Autodesk Inventor part; units mm, degrees
(part 2 of 4)
  spline S241 degree 2 poles (89.3094, 601.3426) (89.3094, 601.1598) (89.3366, 600.9203) (89.3835, 600.8313) knots 0 0 0 1 2 2 2
  spline S242 degree 2 poles (89.3835, 600.8313) (89.4304, 600.7424) (89.591, 600.6609) (89.7416, 600.6609) knots 0 0 0 1 2 2 2
  spline S243 degree 2 poles (89.7416, 600.6609) (89.8824, 600.6609) (90.2011, 600.8215) (90.3345, 600.9375) knots 0 0 0 1 2 2 2
  line L264 (90.3345, 600.9375) -> (90.3345, 602.6468)
  line L265 (90.3345, 602.6468) -> (90.7198, 602.6468)
  line L266 (90.7198, 602.6468) -> (90.7198, 600.3596)
  spline S244 degree 2 poles (91.8955, 600.3052) (91.6658, 600.3052) (91.2681, 600.4287) (91.1372, 600.4979) knots 0 0 0 1 2 2 2
  line L267 (91.1372, 600.4979) -> (91.1372, 600.9301)
  line L268 (91.1372, 600.9301) -> (91.157, 600.9301)
  spline S245 degree 2 poles (91.157, 600.9301) (91.2064, 600.8906) (91.3397, 600.7968) (91.4509, 600.7449) knots 0 0 0 1 2 2 2
  spline S246 degree 2 poles (91.4509, 600.7449) (91.5472, 600.698) (91.7844, 600.6288) (91.9103, 600.6288) knots 0 0 0 1 2 2 2
  spline S247 degree 2 poles (91.9103, 600.6288) (92.0017, 600.6288) (92.2117, 600.6708) (92.2611, 600.7054) knots 0 0 0 1 2 2 2
  spline S248 degree 2 poles (92.2611, 600.7054) (92.3327, 600.7523) (92.3969, 600.8585) (92.3969, 600.9672) knots 0 0 0 1 2 2 2
  spline S249 degree 2 poles (92.3969, 600.9672) (92.3969, 601.103) (92.2487, 601.2438) (92.0585, 601.2908) knots 0 0 0 1 2 2 2
  spline S250 degree 2 poles (92.0585, 601.2908) (91.9844, 601.3081) (91.7473, 601.3575) (91.646, 601.3846) knots 0 0 0 1 2 2 2
  spline S251 degree 2 poles (91.646, 601.3846) (91.3842, 601.4612) (91.1471, 601.7774) (91.1471, 602.0021) knots 0 0 0 1 2 2 2
  spline S252 degree 2 poles (91.1471, 602.0021) (91.1471, 602.3133) (91.6139, 602.7011) (91.9992, 602.7011) knots 0 0 0 1 2 2 2
  spline S253 degree 2 poles (91.9992, 602.7011) (92.1894, 602.7011) (92.5748, 602.6073) (92.7057, 602.5356) knots 0 0 0 1 2 2 2
  line L269 (92.7057, 602.5356) -> (92.7057, 602.1232)
  line L270 (92.7057, 602.1232) -> (92.6859, 602.1232)
  spline S254 degree 2 poles (92.6859, 602.1232) (92.5377, 602.2417) (92.1771, 602.3776) (91.9918, 602.3776) knots 0 0 0 1 2 2 2
  spline S255 degree 2 poles (91.9918, 602.3776) (91.8016, 602.3776) (91.5398, 602.217) (91.5398, 602.0565) knots 0 0 0 1 2 2 2
  spline S256 degree 2 poles (91.5398, 602.0565) (91.5398, 601.9107) (91.6954, 601.7699) (91.8683, 601.7255) knots 0 0 0 1 2 2 2
  spline S257 degree 2 poles (91.8683, 601.7255) (91.9523, 601.7033) (92.1647, 601.6588) (92.2808, 601.6316) knots 0 0 0 1 2 2 2
  spline S258 degree 2 poles (92.2808, 601.6316) (92.5328, 601.5674) (92.7896, 601.2735) (92.7896, 601.0191) knots 0 0 0 1 2 2 2
  spline S259 degree 2 poles (92.7896, 601.0191) (92.7896, 600.8709) (92.6736, 600.609) (92.5599, 600.5127) knots 0 0 0 1 2 2 2
  spline S260 degree 2 poles (92.5599, 600.5127) (92.4389, 600.4114) (92.1302, 600.3052) (91.8955, 600.3052) knots 0 0 0 1 2 2 2
  spline S261 degree 2 poles (93.7653, 600.3052) (93.5356, 600.3052) (93.1379, 600.4287) (93.007, 600.4979) knots 0 0 0 1 2 2 2
  line L271 (93.007, 600.4979) -> (93.007, 600.9301)
  line L272 (93.007, 600.9301) -> (93.0268, 600.9301)
  spline S262 degree 2 poles (93.0268, 600.9301) (93.0762, 600.8906) (93.2095, 600.7968) (93.3207, 600.7449) knots 0 0 0 1 2 2 2
  spline S263 degree 2 poles (93.3207, 600.7449) (93.417, 600.698) (93.6542, 600.6288) (93.7801, 600.6288) knots 0 0 0 1 2 2 2
  spline S264 degree 2 poles (93.7801, 600.6288) (93.8715, 600.6288) (94.0815, 600.6708) (94.1309, 600.7054) knots 0 0 0 1 2 2 2
  spline S265 degree 2 poles (94.1309, 600.7054) (94.2025, 600.7523) (94.2667, 600.8585) (94.2667, 600.9672) knots 0 0 0 1 2 2 2
  spline S266 degree 2 poles (94.2667, 600.9672) (94.2667, 601.103) (94.1185, 601.2438) (93.9283, 601.2908) knots 0 0 0 1 2 2 2
  spline S267 degree 2 poles (93.9283, 601.2908) (93.8542, 601.3081) (93.6171, 601.3575) (93.5158, 601.3846) knots 0 0 0 1 2 2 2
  spline S268 degree 2 poles (93.5158, 601.3846) (93.254, 601.4612) (93.0169, 601.7774) (93.0169, 602.0021) knots 0 0 0 1 2 2 2
  spline S269 degree 2 poles (93.0169, 602.0021) (93.0169, 602.3133) (93.4837, 602.7011) (93.869, 602.7011) knots 0 0 0 1 2 2 2
  spline S270 degree 2 poles (93.869, 602.7011) (94.0592, 602.7011) (94.4446, 602.6073) (94.5755, 602.5356) knots 0 0 0 1 2 2 2
  line L273 (94.5755, 602.5356) -> (94.5755, 602.1232)
  line L274 (94.5755, 602.1232) -> (94.5557, 602.1232)
  spline S271 degree 2 poles (94.5557, 602.1232) (94.4075, 602.2417) (94.0469, 602.3776) (93.8616, 602.3776) knots 0 0 0 1 2 2 2
  spline S272 degree 2 poles (93.8616, 602.3776) (93.6714, 602.3776) (93.4096, 602.217) (93.4096, 602.0565) knots 0 0 0 1 2 2 2
  spline S273 degree 2 poles (93.4096, 602.0565) (93.4096, 601.9107) (93.5652, 601.7699) (93.7381, 601.7255) knots 0 0 0 1 2 2 2
  spline S274 degree 2 poles (93.7381, 601.7255) (93.8221, 601.7033) (94.0345, 601.6588) (94.1506, 601.6316) knots 0 0 0 1 2 2 2
  spline S275 degree 2 poles (94.1506, 601.6316) (94.4026, 601.5674) (94.6594, 601.2735) (94.6594, 601.0191) knots 0 0 0 1 2 2 2
  spline S276 degree 2 poles (94.6594, 601.0191) (94.6594, 600.8709) (94.5434, 600.609) (94.4297, 600.5127) knots 0 0 0 1 2 2 2
  spline S277 degree 2 poles (94.4297, 600.5127) (94.3087, 600.4114) (94, 600.3052) (93.7653, 600.3052) knots 0 0 0 1 2 2 2
  line L275 (95.4103, 600.3596) -> (95.025, 600.3596)
  line L276 (95.025, 600.3596) -> (95.025, 602.6468)
  line L277 (95.025, 602.6468) -> (95.4103, 602.6468)
  line L278 (95.4103, 602.6468) -> (95.4103, 600.3596)
  line L279 (95.4375, 603.0272) -> (95.0003, 603.0272)
  line L280 (95.0003, 603.0272) -> (95.0003, 603.4273)
  line L281 (95.0003, 603.4273) -> (95.4375, 603.4273)
  line L282 (95.4375, 603.4273) -> (95.4375, 603.0272)
  spline S278 degree 2 poles (97.8557, 601.5032) (97.8557, 600.9252) (97.2999, 600.2953) (96.8355, 600.2953) knots 0 0 0 1 2 2 2
  spline S279 degree 2 poles (96.8355, 600.2953) (96.3588, 600.2953) (95.8129, 600.945) (95.8129, 601.5032) knots 0 0 0 1 2 2 2
  spline S280 degree 2 poles (95.8129, 601.5032) (95.8129, 602.0762) (96.3761, 602.711) (96.8355, 602.711) knots 0 0 0 1 2 2 2
  spline S281 degree 2 poles (96.8355, 602.711) (97.2999, 602.711) (97.8557, 602.0787) (97.8557, 601.5032) knots 0 0 0 1 2 2 2
  spline S282 degree 2 poles (97.458, 601.5032) (97.458, 601.9478) (97.1344, 602.38) (96.8355, 602.38) knots 0 0 0 1 2 2 2
  spline S283 degree 2 poles (96.8355, 602.38) (96.5367, 602.38) (96.2106, 601.9478) (96.2106, 601.5032) knots 0 0 0 1 2 2 2
  spline S284 degree 2 poles (96.2106, 601.5032) (96.2106, 601.0709) (96.5367, 600.6263) (96.8355, 600.6263) knots 0 0 0 1 2 2 2
  spline S285 degree 2 poles (96.8355, 600.6263) (97.1319, 600.6263) (97.458, 601.0635) (97.458, 601.5032) knots 0 0 0 1 2 2 2
  line L283 (100.0466, 600.3596) -> (99.6612, 600.3596)
  line L284 (99.6612, 600.3596) -> (99.6612, 601.6637)
  spline S286 degree 2 poles (99.6612, 601.6637) (99.6612, 601.8218) (99.6316, 602.0935) (99.5871, 602.175) knots 0 0 0 1 2 2 2
  spline S287 degree 2 poles (99.5871, 602.175) (99.5402, 602.2615) (99.3722, 602.3455) (99.229, 602.3455) knots 0 0 0 1 2 2 2
  spline S288 degree 2 poles (99.229, 602.3455) (99.0857, 602.3455) (98.7819, 602.1923) (98.6362, 602.0688) knots 0 0 0 1 2 2 2
  line L285 (98.6362, 602.0688) -> (98.6362, 600.3596)
  line L286 (98.6362, 600.3596) -> (98.2509, 600.3596)
  line L287 (98.2509, 600.3596) -> (98.2509, 602.6468)
  line L288 (98.2509, 602.6468) -> (98.6362, 602.6468)
  line L289 (98.6362, 602.6468) -> (98.6362, 602.3924)
  spline S289 degree 2 poles (98.6362, 602.3924) (98.8091, 602.548) (99.1425, 602.711) (99.3302, 602.711) knots 0 0 0 1 2 2 2
  spline S290 degree 2 poles (99.3302, 602.711) (99.6662, 602.711) (100.0466, 602.2664) (100.0466, 601.844) knots 0 0 0 1 2 2 2
  line L290 (100.0466, 601.844) -> (100.0466, 600.3596)
  line L291 (101.6471, 601.5081) -> (100.4936, 601.5081)
  line L292 (100.4936, 601.5081) -> (100.4936, 601.8786)
  line L293 (100.4936, 601.8786) -> (101.6471, 601.8786)
  line L294 (101.6471, 601.8786) -> (101.6471, 601.5081)
  line L295 (104.7519, 600.3596) -> (104.3469, 600.3596)
  line L296 (104.3469, 600.3596) -> (104.3469, 602.9852)
  line L297 (104.3469, 602.9852) -> (103.5515, 601.1994)
  line L298 (103.5515, 601.1994) -> (103.3045, 601.1994)
  line L299 (103.3045, 601.1994) -> (102.5166, 602.9852)
  line L300 (102.5166, 602.9852) -> (102.5166, 600.3596)
  line L301 (102.5166, 600.3596) -> (102.1387, 600.3596)
  line L302 (102.1387, 600.3596) -> (102.1387, 603.4076)
  line L303 (102.1387, 603.4076) -> (102.6919, 603.4076)
  line L304 (102.6919, 603.4076) -> (103.4527, 601.7107)
  line L305 (103.4527, 601.7107) -> (104.1888, 603.4076)
  line L306 (104.1888, 603.4076) -> (104.7519, 603.4076)
  line L307 (104.7519, 603.4076) -> (104.7519, 600.3596)
  spline S291 degree 2 poles (106.6143, 600.6016) (106.5674, 600.567) (106.4093, 600.4435) (106.3352, 600.4065) knots 0 0 0 1 2 2 2
  spline S292 degree 2 poles (106.3352, 600.4065) (106.2339, 600.3522) (106.0438, 600.2953) (105.8709, 600.2953) knots 0 0 0 1 2 2 2
  spline S293 degree 2 poles (105.8709, 600.2953) (105.7301, 600.2953) (105.4757, 600.4016) (105.3793, 600.4979) knots 0 0 0 1 2 2 2
  spline S294 degree 2 poles (105.3793, 600.4979) (105.2879, 600.5917) (105.1768, 600.8684) (105.1768, 601.0215) knots 0 0 0 1 2 2 2
  spline S295 degree 2 poles (105.1768, 601.0215) (105.1768, 601.2587) (105.3768, 601.5946) (105.5942, 601.6909) knots 0 0 0 1 2 2 2
  spline S296 degree 2 poles (105.5942, 601.6909) (105.7869, 601.7798) (106.3105, 601.8465) (106.6143, 601.8638) knots 0 0 0 1 2 2 2
  line L308 (106.6143, 601.8638) -> (106.6143, 601.9379)
  spline S297 degree 2 poles (106.6143, 601.9379) (106.6143, 602.0713) (106.5328, 602.2368) (106.4587, 602.2837) knots 0 0 0 1 2 2 2
  spline S298 degree 2 poles (106.4587, 602.2837) (106.3846, 602.3306) (106.1722, 602.3603) (106.0586, 602.3603) knots 0 0 0 1 2 2 2
  spline S299 degree 2 poles (106.0586, 602.3603) (105.9252, 602.3603) (105.5646, 602.2812) (105.3843, 602.2047) knots 0 0 0 1 2 2 2
  line L309 (105.3843, 602.2047) -> (105.362, 602.2047)
  line L310 (105.362, 602.2047) -> (105.362, 602.5974)
  spline S300 degree 2 poles (105.362, 602.5974) (105.4682, 602.627) (105.8659, 602.7011) (106.061, 602.7011) knots 0 0 0 1 2 2 2
  spline S301 degree 2 poles (106.061, 602.7011) (106.2982, 602.7011) (106.6217, 602.627) (106.7502, 602.5307) knots 0 0 0 1 2 2 2
  spline S302 degree 2 poles (106.7502, 602.5307) (106.8761, 602.4368) (106.9997, 602.138) (106.9997, 601.9231) knots 0 0 0 1 2 2 2
  line L311 (106.9997, 601.9231) -> (106.9997, 600.3596)
  line L312 (106.9997, 600.3596) -> (106.6143, 600.3596)
  line L313 (106.6143, 600.3596) -> (106.6143, 600.6016)
  line L314 (106.6143, 600.9227) -> (106.6143, 601.5575)
  spline S303 degree 2 poles (106.6143, 601.5575) (106.476, 601.5452) (106.0586, 601.5032) (105.9277, 601.4637) knots 0 0 0 1 2 2 2
  spline S304 degree 2 poles (105.9277, 601.4637) (105.7745, 601.4167) (105.5745, 601.2216) (105.5745, 601.0487) knots 0 0 0 1 2 2 2
  spline S305 degree 2 poles (105.5745, 601.0487) (105.5745, 600.8511) (105.7968, 600.651) (106.0092, 600.651) knots 0 0 0 1 2 2 2
  spline S306 degree 2 poles (106.0092, 600.651) (106.1895, 600.651) (106.4859, 600.8066) (106.6143, 600.9227) knots 0 0 0 1 2 2 2
  line L315 (108.7534, 602.2343) -> (108.7336, 602.2343)
  spline S307 degree 2 poles (108.7336, 602.2343) (108.6891, 602.2467) (108.5928, 602.2516) (108.5261, 602.2516) knots 0 0 0 1 2 2 2
  spline S308 degree 2 poles (108.5261, 602.2516) (108.3705, 602.2516) (108.0642, 602.1157) (107.9259, 601.9824) knots 0 0 0 1 2 2 2
  line L316 (107.9259, 601.9824) -> (107.9259, 600.3596)
  line L317 (107.9259, 600.3596) -> (107.5406, 600.3596)
  line L318 (107.5406, 600.3596) -> (107.5406, 602.6468)
  line L319 (107.5406, 602.6468) -> (107.9259, 602.6468)
  line L320 (107.9259, 602.6468) -> (107.9259, 602.3059)
  spline S309 degree 2 poles (107.9259, 602.3059) (108.1359, 602.4937) (108.4495, 602.6468) (108.5978, 602.6468) knots 0 0 0 1 2 2 2
  spline S310 degree 2 poles (108.5978, 602.6468) (108.657, 602.6468) (108.7163, 602.6419) (108.7534, 602.6344) knots 0 0 0 1 2 2 2
  line L321 (108.7534, 602.6344) -> (108.7534, 602.2343)
  spline S311 degree 2 poles (109.9612, 600.3077) (109.7241, 600.3077) (109.3313, 600.4534) (109.1906, 600.6016) knots 0 0 0 1 2 2 2
  spline S312 degree 2 poles (109.1906, 600.6016) (109.0498, 600.7474) (108.8942, 601.1969) (108.8942, 601.4982) knots 0 0 0 1 2 2 2
  spline S313 degree 2 poles (108.8942, 601.4982) (108.8942, 601.7996) (109.0547, 602.2392) (109.1906, 602.3874) knots 0 0 0 1 2 2 2
  spline S314 degree 2 poles (109.1906, 602.3874) (109.3264, 602.5381) (109.729, 602.6987) (109.9612, 602.6987) knots 0 0 0 1 2 2 2
  spline S315 degree 2 poles (109.9612, 602.6987) (110.1489, 602.6987) (110.4997, 602.5925) (110.6355, 602.5233) knots 0 0 0 1 2 2 2
  line L322 (110.6355, 602.5233) -> (110.6355, 602.091)
  line L323 (110.6355, 602.091) -> (110.6133, 602.091)
  spline S316 degree 2 poles (110.6133, 602.091) (110.5713, 602.1256) (110.4429, 602.2145) (110.3515, 602.2615) knots 0 0 0 1 2 2 2
  spline S317 degree 2 poles (110.3515, 602.2615) (110.27, 602.301) (110.0526, 602.3627) (109.9538, 602.3627) knots 0 0 0 1 2 2 2
  spline S318 degree 2 poles (109.9538, 602.3627) (109.6549, 602.3627) (109.2918, 601.9107) (109.2918, 601.4982) knots 0 0 0 1 2 2 2
  spline S319 degree 2 poles (109.2918, 601.4982) (109.2918, 601.0956) (109.6426, 600.6436) (109.9538, 600.6436) knots 0 0 0 1 2 2 2
  spline S320 degree 2 poles (109.9538, 600.6436) (110.1415, 600.6436) (110.4824, 600.7992) (110.6133, 600.9203) knots 0 0 0 1 2 2 2
  line L324 (110.6133, 600.9203) -> (110.6355, 600.9203)
  line L325 (110.6355, 600.9203) -> (110.6355, 600.488)
  spline S321 degree 2 poles (110.6355, 600.488) (110.5787, 600.4608) (110.4058, 600.3843) (110.3366, 600.367) knots 0 0 0 1 2 2 2
  spline S322 degree 2 poles (110.3366, 600.367) (110.2378, 600.3373) (110.0822, 600.3077) (109.9612, 600.3077) knots 0 0 0 1 2 2 2
  line L326 (112.782, 600.3596) -> (112.3966, 600.3596)
  line L327 (112.3966, 600.3596) -> (112.3966, 601.6637)
  spline S323 degree 2 poles (112.3966, 601.6637) (112.3966, 601.8218) (112.367, 602.0935) (112.3225, 602.175) knots 0 0 0 1 2 2 2
  spline S324 degree 2 poles (112.3225, 602.175) (112.2756, 602.2615) (112.1076, 602.3455) (111.9644, 602.3455) knots 0 0 0 1 2 2 2
  spline S325 degree 2 poles (111.9644, 602.3455) (111.8211, 602.3455) (111.5173, 602.1923) (111.3716, 602.0688) knots 0 0 0 1 2 2 2
  line L328 (111.3716, 602.0688) -> (111.3716, 600.3596)
  line L329 (111.3716, 600.3596) -> (110.9863, 600.3596)
  line L330 (110.9863, 600.3596) -> (110.9863, 603.5434)
  line L331 (110.9863, 603.5434) -> (111.3716, 603.5434)
  line L332 (111.3716, 603.5434) -> (111.3716, 602.3924)
  spline S326 degree 2 poles (111.3716, 602.3924) (111.5445, 602.548) (111.8779, 602.711) (112.0657, 602.711) knots 0 0 0 1 2 2 2
  spline S327 degree 2 poles (112.0657, 602.711) (112.4016, 602.711) (112.782, 602.2664) (112.782, 601.844) knots 0 0 0 1 2 2 2
  line L333 (112.782, 601.844) -> (112.782, 600.3596)
  line L334 (113.7156, 600.3596) -> (113.3303, 600.3596)
  line L335 (113.3303, 600.3596) -> (113.3303, 602.6468)
  line L336 (113.3303, 602.6468) -> (113.7156, 602.6468)
  line L337 (113.7156, 602.6468) -> (113.7156, 600.3596)
  line L338 (113.7428, 603.0272) -> (113.3056, 603.0272)
  line L339 (113.3056, 603.0272) -> (113.3056, 603.4273)
  line L340 (113.3056, 603.4273) -> (113.7428, 603.4273)
  line L341 (113.7428, 603.4273) -> (113.7428, 603.0272)
  line L342 (116.077, 600.3596) -> (115.6916, 600.3596)
  line L343 (115.6916, 600.3596) -> (115.6916, 601.6637)
  spline S328 degree 2 poles (115.6916, 601.6637) (115.6916, 601.8218) (115.662, 602.0935) (115.6175, 602.175) knots 0 0 0 1 2 2 2
  spline S329 degree 2 poles (115.6175, 602.175) (115.5706, 602.2615) (115.4026, 602.3455) (115.2594, 602.3455) knots 0 0 0 1 2 2 2
  spline S330 degree 2 poles (115.2594, 602.3455) (115.1161, 602.3455) (114.8123, 602.1923) (114.6666, 602.0688) knots 0 0 0 1 2 2 2
  line L344 (114.6666, 602.0688) -> (114.6666, 600.3596)
  line L345 (114.6666, 600.3596) -> (114.2813, 600.3596)
  line L346 (114.2813, 600.3596) -> (114.2813, 602.6468)
  line L347 (114.2813, 602.6468) -> (114.6666, 602.6468)
  line L348 (114.6666, 602.6468) -> (114.6666, 602.3924)
  spline S331 degree 2 poles (114.6666, 602.3924) (114.8395, 602.548) (115.1729, 602.711) (115.3607, 602.711) knots 0 0 0 1 2 2 2
  spline S332 degree 2 poles (115.3607, 602.711) (115.6966, 602.711) (116.077, 602.2664) (116.077, 601.844) knots 0 0 0 1 2 2 2
  line L349 (116.077, 601.844) -> (116.077, 600.3596)
  spline S333 degree 2 poles (116.6994, 599.994) (116.7389, 599.9767) (116.8896, 599.9224) (116.9859, 599.9001) knots 0 0 0 1 2 2 2
  spline S334 degree 2 poles (116.9859, 599.9001) (117.0921, 599.873) (117.2724, 599.8409) (117.3787, 599.8409) knots 0 0 0 1 2 2 2
  spline S335 degree 2 poles (117.3787, 599.8409) (117.5565, 599.8409) (117.8035, 599.9347) (117.8727, 600.0187) knots 0 0 0 1 2 2 2
  spline S336 degree 2 poles (117.8727, 600.0187) (117.9394, 600.1027) (117.9912, 600.3225) (117.9912, 600.4633) knots 0 0 0 1 2 2 2
  line L350 (117.9912, 600.4633) -> (117.9912, 600.6634)
  spline S337 degree 2 poles (117.9912, 600.6634) (117.8356, 600.5275) (117.5367, 600.3991) (117.312, 600.3991) knots 0 0 0 1 2 2 2
  spline S338 degree 2 poles (117.312, 600.3991) (116.9217, 600.3991) (116.4598, 600.9795) (116.4598, 601.5254) knots 0 0 0 1 2 2 2
  spline S339 degree 2 poles (116.4598, 601.5254) (116.4598, 601.8095) (116.6204, 602.2491) (116.7537, 602.4047) knots 0 0 0 1 2 2 2
  spline S340 degree 2 poles (116.7537, 602.4047) (116.8822, 602.5505) (117.2354, 602.711) (117.4231, 602.711) knots 0 0 0 1 2 2 2
  spline S341 degree 2 poles (117.4231, 602.711) (117.601, 602.711) (117.8603, 602.627) (117.9912, 602.5505) knots 0 0 0 1 2 2 2
  line L351 (117.9912, 602.5505) -> (118.0135, 602.6468)
  line L352 (118.0135, 602.6468) -> (118.3765, 602.6468)
  line L353 (118.3765, 602.6468) -> (118.3765, 600.6214)
  spline S342 degree 2 poles (118.3765, 600.6214) (118.3765, 600.0385) (117.8702, 599.4951) (117.349, 599.4951) knots 0 0 0 1 2 2 2
  spline S343 degree 2 poles (117.349, 599.4951) (117.1811, 599.4951) (116.8303, 599.5494) (116.6796, 599.5939) knots 0 0 0 1 2 2 2
  line L354 (116.6796, 599.5939) -> (116.6796, 599.994)
  line L355 (116.6796, 599.994) -> (116.6994, 599.994)
  line L356 (117.9912, 600.9795) -> (117.9912, 602.2368)
  spline S344 degree 2 poles (117.9912, 602.2368) (117.848, 602.3059) (117.6059, 602.3652) (117.4849, 602.3652) knots 0 0 0 1 2 2 2
  spline S345 degree 2 poles (117.4849, 602.3652) (117.1934, 602.3652) (116.8575, 601.9354) (116.8575, 601.5328) knots 0 0 0 1 2 2 2
  spline S346 degree 2 poles (116.8575, 601.5328) (116.8575, 601.1524) (117.1119, 600.7548) (117.3984, 600.7548) knots 0 0 0 1 2 2 2
  spline S347 degree 2 poles (117.3984, 600.7548) (117.5491, 600.7548) (117.8653, 600.8733) (117.9912, 600.9795) knots 0 0 0 1 2 2 2
  line L357 (119.9944, 601.5081) -> (118.8409, 601.5081)
  line L358 (118.8409, 601.5081) -> (118.8409, 601.8786)
  line L359 (118.8409, 601.8786) -> (119.9944, 601.8786)
  line L360 (119.9944, 601.8786) -> (119.9944, 601.5081)
  spline S348 degree 2 poles (121.6765, 600.3052) (121.3801, 600.3052) (120.8787, 600.5053) (120.6959, 600.7054) knots 0 0 0 1 2 2 2
  spline S349 degree 2 poles (120.6959, 600.7054) (120.5131, 600.903) (120.313, 601.4958) (120.313, 601.8811) knots 0 0 0 1 2 2 2
  spline S350 degree 2 poles (120.313, 601.8811) (120.313, 602.2639) (120.5082, 602.8321) (120.6934, 603.042) knots 0 0 0 1 2 2 2
  spline S351 degree 2 poles (120.6934, 603.042) (120.8762, 603.247) (121.3751, 603.4619) (121.6839, 603.4619) knots 0 0 0 1 2 2 2
  spline S352 degree 2 poles (121.6839, 603.4619) (121.837, 603.4619) (122.1063, 603.4174) (122.2199, 603.3829) knots 0 0 0 1 2 2 2
  spline S353 degree 2 poles (122.2199, 603.3829) (122.3187, 603.3508) (122.5237, 603.2594) (122.625, 603.205) knots 0 0 0 1 2 2 2
  line L361 (122.625, 603.205) -> (122.625, 602.716)
  line L362 (122.625, 602.716) -> (122.5929, 602.716)
  spline S354 degree 2 poles (122.5929, 602.716) (122.5385, 602.7654) (122.3706, 602.9037) (122.2495, 602.9704) knots 0 0 0 1 2 2 2
  spline S355 degree 2 poles (122.2495, 602.9704) (122.1334, 603.0346) (121.8593, 603.1161) (121.6814, 603.1161) knots 0 0 0 1 2 2 2
  spline S356 degree 2 poles (121.6814, 603.1161) (121.4863, 603.1161) (121.138, 602.9556) (121.0071, 602.8024) knots 0 0 0 1 2 2 2
  spline S357 degree 2 poles (121.0071, 602.8024) (120.8787, 602.6468) (120.7354, 602.175) (120.7354, 601.8811) knots 0 0 0 1 2 2 2
  spline S358 degree 2 poles (120.7354, 601.8811) (120.7354, 601.5674) (120.8861, 601.1154) (121.017, 600.9598) knots 0 0 0 1 2 2 2
  spline S359 degree 2 poles (121.017, 600.9598) (121.1454, 600.8091) (121.4888, 600.656) (121.6814, 600.656) knots 0 0 0 1 2 2 2
  spline S360 degree 2 poles (121.6814, 600.656) (121.8568, 600.656) (122.1557, 600.7424) (122.2718, 600.8066) knots 0 0 0 1 2 2 2
  spline S361 degree 2 poles (122.2718, 600.8066) (122.3829, 600.8709) (122.5484, 601.0042) (122.5953, 601.0512) knots 0 0 0 1 2 2 2
  line L363 (122.5953, 601.0512) -> (122.625, 601.0512)
  line L364 (122.625, 601.0512) -> (122.625, 600.567)
  spline S362 degree 2 poles (122.625, 600.567) (122.5237, 600.5201) (122.3459, 600.4337) (122.2199, 600.3941) knots 0 0 0 1 2 2 2
  spline S363 degree 2 poles (122.2199, 600.3941) (122.0865, 600.3497) (121.8593, 600.3052) (121.6765, 600.3052) knots 0 0 0 1 2 2 2
  spline S364 degree 2 poles (124.2478, 600.6016) (124.2008, 600.567) (124.0428, 600.4435) (123.9687, 600.4065) knots 0 0 0 1 2 2 2
  spline S365 degree 2 poles (123.9687, 600.4065) (123.8674, 600.3522) (123.6772, 600.2953) (123.5043, 600.2953) knots 0 0 0 1 2 2 2
  spline S366 degree 2 poles (123.5043, 600.2953) (123.3635, 600.2953) (123.1091, 600.4016) (123.0128, 600.4979) knots 0 0 0 1 2 2 2
  spline S367 degree 2 poles (123.0128, 600.4979) (122.9214, 600.5917) (122.8102, 600.8684) (122.8102, 601.0215) knots 0 0 0 1 2 2 2
  spline S368 degree 2 poles (122.8102, 601.0215) (122.8102, 601.2587) (123.0103, 601.5946) (123.2277, 601.6909) knots 0 0 0 1 2 2 2
  spline S369 degree 2 poles (123.2277, 601.6909) (123.4203, 601.7798) (123.944, 601.8465) (124.2478, 601.8638) knots 0 0 0 1 2 2 2
  line L365 (124.2478, 601.8638) -> (124.2478, 601.9379)
  spline S370 degree 2 poles (124.2478, 601.9379) (124.2478, 602.0713) (124.1663, 602.2368) (124.0922, 602.2837) knots 0 0 0 1 2 2 2
  spline S371 degree 2 poles (124.0922, 602.2837) (124.0181, 602.3306) (123.8056, 602.3603) (123.692, 602.3603) knots 0 0 0 1 2 2 2
  spline S372 degree 2 poles (123.692, 602.3603) (123.5586, 602.3603) (123.198, 602.2812) (123.0177, 602.2047) knots 0 0 0 1 2 2 2
  line L366 (123.0177, 602.2047) -> (122.9955, 602.2047)
  line L367 (122.9955, 602.2047) -> (122.9955, 602.5974)
  spline S373 degree 2 poles (122.9955, 602.5974) (123.1017, 602.627) (123.4994, 602.7011) (123.6945, 602.7011) knots 0 0 0 1 2 2 2
  spline S374 degree 2 poles (123.6945, 602.7011) (123.9316, 602.7011) (124.2552, 602.627) (124.3836, 602.5307) knots 0 0 0 1 2 2 2
  spline S375 degree 2 poles (124.3836, 602.5307) (124.5096, 602.4368) (124.6331, 602.138) (124.6331, 601.9231) knots 0 0 0 1 2 2 2
  line L368 (124.6331, 601.9231) -> (124.6331, 600.3596)
  line L369 (124.6331, 600.3596) -> (124.2478, 600.3596)
  line L370 (124.2478, 600.3596) -> (124.2478, 600.6016)
  line L371 (124.2478, 600.9227) -> (124.2478, 601.5575)
  spline S376 degree 2 poles (124.2478, 601.5575) (124.1095, 601.5452) (123.692, 601.5032) (123.5611, 601.4637) knots 0 0 0 1 2 2 2
  spline S377 degree 2 poles (123.5611, 601.4637) (123.408, 601.4167) (123.2079, 601.2216) (123.2079, 601.0487) knots 0 0 0 1 2 2 2
  spline S378 degree 2 poles (123.2079, 601.0487) (123.2079, 600.8511) (123.4302, 600.651) (123.6426, 600.651) knots 0 0 0 1 2 2 2
  spline S379 degree 2 poles (123.6426, 600.651) (123.8229, 600.651) (124.1193, 600.8066) (124.2478, 600.9227) knots 0 0 0 1 2 2 2
  line L372 (126.3868, 602.2343) -> (126.367, 602.2343)
  spline S380 degree 2 poles (126.367, 602.2343) (126.3226, 602.2467) (126.2263, 602.2516) (126.1596, 602.2516) knots 0 0 0 1 2 2 2
  spline S381 degree 2 poles (126.1596, 602.2516) (126.004, 602.2516) (125.6977, 602.1157) (125.5594, 601.9824) knots 0 0 0 1 2 2 2
  line L373 (125.5594, 601.9824) -> (125.5594, 600.3596)
  line L374 (125.5594, 600.3596) -> (125.174, 600.3596)
  line L375 (125.174, 600.3596) -> (125.174, 602.6468)
  line L376 (125.174, 602.6468) -> (125.5594, 602.6468)
  line L377 (125.5594, 602.6468) -> (125.5594, 602.3059)
  spline S382 degree 2 poles (125.5594, 602.3059) (125.7693, 602.4937) (126.083, 602.6468) (126.2312, 602.6468) knots 0 0 0 1 2 2 2
  spline S383 degree 2 poles (126.2312, 602.6468) (126.2905, 602.6468) (126.3498, 602.6419) (126.3868, 602.6344) knots 0 0 0 1 2 2 2
  line L378 (126.3868, 602.6344) -> (126.3868, 602.2343)
  line L379 (127.8985, 602.2343) -> (127.8787, 602.2343)
  spline S384 degree 2 poles (127.8787, 602.2343) (127.8342, 602.2467) (127.7379, 602.2516) (127.6712, 602.2516) knots 0 0 0 1 2 2 2
  spline S385 degree 2 poles (127.6712, 602.2516) (127.5156, 602.2516) (127.2093, 602.1157) (127.071, 601.9824) knots 0 0 0 1 2 2 2
  line L380 (127.071, 601.9824) -> (127.071, 600.3596)
  line L381 (127.071, 600.3596) -> (126.6857, 600.3596)
  line L382 (126.6857, 600.3596) -> (126.6857, 602.6468)
  line L383 (126.6857, 602.6468) -> (127.071, 602.6468)
  line L384 (127.071, 602.6468) -> (127.071, 602.3059)
  spline S386 degree 2 poles (127.071, 602.3059) (127.281, 602.4937) (127.5946, 602.6468) (127.7428, 602.6468) knots 0 0 0 1 2 2 2
  spline S387 degree 2 poles (127.7428, 602.6468) (127.8021, 602.6468) (127.8614, 602.6419) (127.8985, 602.6344) knots 0 0 0 1 2 2 2
  line L385 (127.8985, 602.6344) -> (127.8985, 602.2343)
  line L386 (128.5901, 600.3596) -> (128.2047, 600.3596)
  line L387 (128.2047, 600.3596) -> (128.2047, 602.6468)
  line L388 (128.2047, 602.6468) -> (128.5901, 602.6468)
  line L389 (128.5901, 602.6468) -> (128.5901, 600.3596)
  line L390 (128.6172, 603.0272) -> (128.18, 603.0272)
  line L391 (128.18, 603.0272) -> (128.18, 603.4273)
  line L392 (128.18, 603.4273) -> (128.6172, 603.4273)
  line L393 (128.6172, 603.4273) -> (128.6172, 603.0272)
  spline S388 degree 2 poles (130.1486, 600.3077) (129.6003, 600.3077) (128.9976, 600.9227) (128.9976, 601.4908) knots 0 0 0 1 2 2 2
  spline S389 degree 2 poles (128.9976, 601.4908) (128.9976, 602.0491) (129.583, 602.711) (130.0548, 602.711) knots 0 0 0 1 2 2 2
  spline S390 degree 2 poles (130.0548, 602.711) (130.2672, 602.711) (130.5957, 602.5875) (130.7167, 602.4566) knots 0 0 0 1 2 2 2
  spline S391 degree 2 poles (130.7167, 602.4566) (130.8402, 602.3257) (130.9712, 601.9478) (130.9712, 601.6736) knots 0 0 0 1 2 2 2
  line L394 (130.9712, 601.6736) -> (130.9712, 601.4637)
  line L395 (130.9712, 601.4637) -> (129.3879, 601.4637)
  spline S392 degree 2 poles (129.3879, 601.4637) (129.3879, 601.066) (129.788, 600.6436) (130.1437, 600.6436) knots 0 0 0 1 2 2 2
  spline S393 degree 2 poles (130.1437, 600.6436) (130.2697, 600.6436) (130.5142, 600.7004) (130.613, 600.7449) knots 0 0 0 1 2 2 2
  spline S394 degree 2 poles (130.613, 600.7449) (130.7167, 600.7943) (130.86, 600.8807) (130.9069, 600.9203) knots 0 0 0 1 2 2 2
  line L396 (130.9069, 600.9203) -> (130.9292, 600.9203)
  line L397 (130.9292, 600.9203) -> (130.9292, 600.5004)
  spline S395 degree 2 poles (130.9292, 600.5004) (130.8625, 600.4732) (130.6599, 600.3941) (130.5809, 600.3719) knots 0 0 0 1 2 2 2
  spline S396 degree 2 poles (130.5809, 600.3719) (130.4697, 600.3398) (130.287, 600.3077) (130.1486, 600.3077) knots 0 0 0 1 2 2 2
  spline S397 degree 2 poles (130.5957, 601.7576) (130.5908, 601.9132) (130.5266, 602.1404) (130.4648, 602.217) knots 0 0 0 1 2 2 2
  spline S398 degree 2 poles (130.4648, 602.217) (130.3981, 602.3035) (130.1882, 602.3949) (130.0326, 602.3949) knots 0 0 0 1 2 2 2
  spline S399 degree 2 poles (130.0326, 602.3949) (129.8794, 602.3949) (129.6645, 602.3035) (129.5756, 602.2145) knots 0 0 0 1 2 2 2
  spline S400 degree 2 poles (129.5756, 602.2145) (129.4891, 602.1232) (129.4002, 601.9033) (129.3879, 601.7576) knots 0 0 0 1 2 2 2
  line L398 (129.3879, 601.7576) -> (130.5957, 601.7576)
  line L399 (132.5742, 602.2343) -> (132.5544, 602.2343)
  spline S401 degree 2 poles (132.5544, 602.2343) (132.51, 602.2467) (132.4136, 602.2516) (132.347, 602.2516) knots 0 0 0 1 2 2 2
  spline S402 degree 2 poles (132.347, 602.2516) (132.1913, 602.2516) (131.8851, 602.1157) (131.7467, 601.9824) knots 0 0 0 1 2 2 2
  line L400 (131.7467, 601.9824) -> (131.7467, 600.3596)
  line L401 (131.7467, 600.3596) -> (131.3614, 600.3596)
  line L402 (131.3614, 600.3596) -> (131.3614, 602.6468)
  line L403 (131.3614, 602.6468) -> (131.7467, 602.6468)
  line L404 (131.7467, 602.6468) -> (131.7467, 602.3059)
  spline S403 degree 2 poles (131.7467, 602.3059) (131.9567, 602.4937) (132.2704, 602.6468) (132.4186, 602.6468) knots 0 0 0 1 2 2 2
  spline S404 degree 2 poles (132.4186, 602.6468) (132.4779, 602.6468) (132.5371, 602.6419) (132.5742, 602.6344) knots 0 0 0 1 2 2 2
  line L405 (132.5742, 602.6344) -> (132.5742, 602.2343)
  line L406 (133.9327, 601.5081) -> (132.7792, 601.5081)
  line L407 (132.7792, 601.5081) -> (132.7792, 601.8786)
  line L408 (132.7792, 601.8786) -> (133.9327, 601.8786)
  line L409 (133.9327, 601.8786) -> (133.9327, 601.5081)
  spline S405 degree 2 poles (135.2739, 600.3052) (134.9429, 600.3052) (134.4786, 600.4435) (134.2736, 600.5423) knots 0 0 0 1 2 2 2
  line L410 (134.2736, 600.5423) -> (134.2736, 601.0512)
  line L411 (134.2736, 601.0512) -> (134.3032, 601.0512)
  spline S406 degree 2 poles (134.3032, 601.0512) (134.5033, 600.8634) (135.0096, 600.656) (135.2443, 600.656) knots 0 0 0 1 2 2 2
  spline S407 degree 2 poles (135.2443, 600.656) (135.5802, 600.656) (135.9235, 600.9351) (135.9235, 601.1648) knots 0 0 0 1 2 2 2
  spline S408 degree 2 poles (135.9235, 601.1648) (135.9235, 601.3476) (135.7432, 601.5748) (135.5481, 601.6316) knots 0 0 0 1 2 2 2
  spline S409 degree 2 poles (135.5481, 601.6316) (135.4073, 601.6711) (135.1727, 601.7255) (134.9973, 601.7699) knots 0 0 0 1 2 2 2
  spline S410 degree 2 poles (134.9973, 601.7699) (134.8392, 601.8119) (134.5897, 601.9379) (134.4934, 602.0392) knots 0 0 0 1 2 2 2
  spline S411 degree 2 poles (134.4934, 602.0392) (134.3995, 602.1404) (134.2958, 602.4121) (134.2958, 602.59) knots 0 0 0 1 2 2 2
  spline S412 degree 2 poles (134.2958, 602.59) (134.2958, 602.9605) (134.8738, 603.4619) (135.3209, 603.4619) knots 0 0 0 1 2 2 2
  spline S413 degree 2 poles (135.3209, 603.4619) (135.5777, 603.4619) (136.0322, 603.3606) (136.2274, 603.2643) knots 0 0 0 1 2 2 2
  line L412 (136.2274, 603.2643) -> (136.2274, 602.7802)
  line L413 (136.2274, 602.7802) -> (136.1977, 602.7802)
  spline S414 degree 2 poles (136.1977, 602.7802) (136.052, 602.9136) (135.5975, 603.1112) (135.348, 603.1112) knots 0 0 0 1 2 2 2
  spline S415 degree 2 poles (135.348, 603.1112) (135.0664, 603.1112) (134.7182, 602.8469) (134.7182, 602.632) knots 0 0 0 1 2 2 2
  spline S416 degree 2 poles (134.7182, 602.632) (134.7182, 602.4393) (134.9232, 602.2096) (135.1158, 602.1577) knots 0 0 0 1 2 2 2
  spline S417 degree 2 poles (135.1158, 602.1577) (135.2443, 602.1232) (135.6173, 602.0342) (135.7408, 601.9972) knots 0 0 0 1 2 2 2
  spline S418 degree 2 poles (135.7408, 601.9972) (136.0545, 601.9009) (136.3459, 601.5131) (136.3459, 601.229) knots 0 0 0 1 2 2 2
  spline S419 degree 2 poles (136.3459, 601.229) (136.3459, 601.0487) (136.2002, 600.7029) (136.0693, 600.5819) knots 0 0 0 1 2 2 2
  spline S420 degree 2 poles (136.0693, 600.5819) (135.9235, 600.4485) (135.553, 600.3052) (135.2739, 600.3052) knots 0 0 0 1 2 2 2
  line L414 (138.5245, 600.3596) -> (138.1391, 600.3596)
  line L415 (138.1391, 600.3596) -> (138.1391, 601.6637)
  spline S421 degree 2 poles (138.1391, 601.6637) (138.1391, 601.8218) (138.1095, 602.0935) (138.065, 602.175) knots 0 0 0 1 2 2 2
  spline S422 degree 2 poles (138.065, 602.175) (138.0181, 602.2615) (137.8502, 602.3455) (137.7069, 602.3455) knots 0 0 0 1 2 2 2
  spline S423 degree 2 poles (137.7069, 602.3455) (137.5636, 602.3455) (137.2598, 602.1923) (137.1141, 602.0688) knots 0 0 0 1 2 2 2
  line L416 (137.1141, 602.0688) -> (137.1141, 600.3596)
  line L417 (137.1141, 600.3596) -> (136.7288, 600.3596)
  line L418 (136.7288, 600.3596) -> (136.7288, 603.5434)
  line L419 (136.7288, 603.5434) -> (137.1141, 603.5434)
  line L420 (137.1141, 603.5434) -> (137.1141, 602.3924)
  spline S424 degree 2 poles (137.1141, 602.3924) (137.287, 602.548) (137.6204, 602.711) (137.8082, 602.711) knots 0 0 0 1 2 2 2
  spline S425 degree 2 poles (137.8082, 602.711) (138.1441, 602.711) (138.5245, 602.2664) (138.5245, 601.844) knots 0 0 0 1 2 2 2
  line L421 (138.5245, 601.844) -> (138.5245, 600.3596)
  spline S426 degree 2 poles (140.9451, 601.5032) (140.9451, 600.9252) (140.3893, 600.2953) (139.925, 600.2953) knots 0 0 0 1 2 2 2
  spline S427 degree 2 poles (139.925, 600.2953) (139.4483, 600.2953) (138.9024, 600.945) (138.9024, 601.5032) knots 0 0 0 1 2 2 2
  spline S428 degree 2 poles (138.9024, 601.5032) (138.9024, 602.0762) (139.4655, 602.711) (139.925, 602.711) knots 0 0 0 1 2 2 2
  spline S429 degree 2 poles (139.925, 602.711) (140.3893, 602.711) (140.9451, 602.0787) (140.9451, 601.5032) knots 0 0 0 1 2 2 2
  spline S430 degree 2 poles (140.5474, 601.5032) (140.5474, 601.9478) (140.2238, 602.38) (139.925, 602.38) knots 0 0 0 1 2 2 2
  spline S431 degree 2 poles (139.925, 602.38) (139.6261, 602.38) (139.3001, 601.9478) (139.3001, 601.5032) knots 0 0 0 1 2 2 2
  spline S432 degree 2 poles (139.3001, 601.5032) (139.3001, 601.0709) (139.6261, 600.6263) (139.925, 600.6263) knots 0 0 0 1 2 2 2
  spline S433 degree 2 poles (139.925, 600.6263) (140.2214, 600.6263) (140.5474, 601.0635) (140.5474, 601.5032) knots 0 0 0 1 2 2 2
  line L422 (143.1187, 600.3596) -> (142.7334, 600.3596)
  line L423 (142.7334, 600.3596) -> (142.7334, 600.6115)
  spline S434 degree 2 poles (142.7334, 600.6115) (142.5555, 600.4559) (142.2369, 600.2953) (142.0393, 600.2953) knots 0 0 0 1 2 2 2
  spline S435 degree 2 poles (142.0393, 600.2953) (141.8911, 600.2953) (141.6268, 600.3941) (141.5305, 600.5004) knots 0 0 0 1 2 2 2
  spline S436 degree 2 poles (141.5305, 600.5004) (141.4317, 600.6066) (141.323, 600.9301) (141.323, 601.1623) knots 0 0 0 1 2 2 2
  line L424 (141.323, 601.1623) -> (141.323, 602.6468)
  line L425 (141.323, 602.6468) -> (141.7083, 602.6468)
  line L426 (141.7083, 602.6468) -> (141.7083, 601.3426)
  spline S437 degree 2 poles (141.7083, 601.3426) (141.7083, 601.1598) (141.7355, 600.9203) (141.7824, 600.8313) knots 0 0 0 1 2 2 2
  spline S438 degree 2 poles (141.7824, 600.8313) (141.8293, 600.7424) (141.9899, 600.6609) (142.1406, 600.6609) knots 0 0 0 1 2 2 2
  spline S439 degree 2 poles (142.1406, 600.6609) (142.2814, 600.6609) (142.6, 600.8215) (142.7334, 600.9375) knots 0 0 0 1 2 2 2
  line L427 (142.7334, 600.9375) -> (142.7334, 602.6468)
  line L428 (142.7334, 602.6468) -> (143.1187, 602.6468)
  line L429 (143.1187, 602.6468) -> (143.1187, 600.3596)
  line L430 (144.0697, 600.3596) -> (143.6843, 600.3596)
  line L431 (143.6843, 600.3596) -> (143.6843, 603.5434)
  line L432 (143.6843, 603.5434) -> (144.0697, 603.5434)
  line L433 (144.0697, 603.5434) -> (144.0697, 600.3596)
  line L434 (146.3939, 600.3596) -> (146.0086, 600.3596)
  line L435 (146.0086, 600.3596) -> (146.0086, 600.5917)
  spline S440 degree 2 poles (146.0086, 600.5917) (145.9197, 600.5176) (145.7888, 600.4188) (145.6999, 600.3769) knots 0 0 0 1 2 2 2
  spline S441 degree 2 poles (145.6999, 600.3769) (145.6184, 600.3373) (145.443, 600.2953) (145.3269, 600.2953) knots 0 0 0 1 2 2 2
  spline S442 degree 2 poles (145.3269, 600.2953) (145.1392, 600.2953) (144.823, 600.451) (144.7119, 600.6016) knots 0 0 0 1 2 2 2
  spline S443 degree 2 poles (144.7119, 600.6016) (144.6007, 600.7523) (144.4772, 601.1969) (144.4772, 601.4859) knots 0 0 0 1 2 2 2
  spline S444 degree 2 poles (144.4772, 601.4859) (144.4772, 601.7872) (144.6328, 602.2269) (144.7687, 602.3924) knots 0 0 0 1 2 2 2
  spline S445 degree 2 poles (144.7687, 602.3924) (144.8946, 602.5406) (145.2479, 602.711) (145.443, 602.711) knots 0 0 0 1 2 2 2
  spline S446 degree 2 poles (145.443, 602.711) (145.6134, 602.711) (145.8678, 602.6344) (146.0086, 602.5554) knots 0 0 0 1 2 2 2
  line L436 (146.0086, 602.5554) -> (146.0086, 603.5434)
  line L437 (146.0086, 603.5434) -> (146.3939, 603.5434)
  line L438 (146.3939, 603.5434) -> (146.3939, 600.3596)
  line L439 (146.0086, 600.9153) -> (146.0086, 602.2368)
  spline S447 degree 2 poles (146.0086, 602.2368) (145.8654, 602.3059) (145.6381, 602.3578) (145.5072, 602.3578) knots 0 0 0 1 2 2 2
  spline S448 degree 2 poles (145.5072, 602.3578) (145.2108, 602.3578) (144.8749, 601.9132) (144.8749, 601.4933) knots 0 0 0 1 2 2 2
  spline S449 degree 2 poles (144.8749, 601.4933) (144.8749, 601.0882) (145.1318, 600.6609) (145.4158, 600.6609) knots 0 0 0 1 2 2 2
  spline S450 degree 2 poles (145.4158, 600.6609) (145.5665, 600.6609) (145.8728, 600.7992) (146.0086, 600.9153) knots 0 0 0 1 2 2 2
  spline S451 degree 2 poles (147.9451, 600.3077) (147.3968, 600.3077) (146.7941, 600.9227) (146.7941, 601.4908) knots 0 0 0 1 2 2 2
  spline S452 degree 2 poles (146.7941, 601.4908) (146.7941, 602.0491) (147.3795, 602.711) (147.8512, 602.711) knots 0 0 0 1 2 2 2
  spline S453 degree 2 poles (147.8512, 602.711) (148.0637, 602.711) (148.3922, 602.5875) (148.5132, 602.4566) knots 0 0 0 1 2 2 2
  spline S454 degree 2 poles (148.5132, 602.4566) (148.6367, 602.3257) (148.7676, 601.9478) (148.7676, 601.6736) knots 0 0 0 1 2 2 2
  line L440 (148.7676, 601.6736) -> (148.7676, 601.4637)
  line L441 (148.7676, 601.4637) -> (147.1843, 601.4637)
  spline S455 degree 2 poles (147.1843, 601.4637) (147.1843, 601.066) (147.5845, 600.6436) (147.9402, 600.6436) knots 0 0 0 1 2 2 2
  spline S456 degree 2 poles (147.9402, 600.6436) (148.0661, 600.6436) (148.3107, 600.7004) (148.4095, 600.7449) knots 0 0 0 1 2 2 2
  spline S457 degree 2 poles (148.4095, 600.7449) (148.5132, 600.7943) (148.6565, 600.8807) (148.7034, 600.9203) knots 0 0 0 1 2 2 2
  line L442 (148.7034, 600.9203) -> (148.7256, 600.9203)
  line L443 (148.7256, 600.9203) -> (148.7256, 600.5004)
  spline S458 degree 2 poles (148.7256, 600.5004) (148.6589, 600.4732) (148.4564, 600.3941) (148.3774, 600.3719) knots 0 0 0 1 2 2 2
  spline S459 degree 2 poles (148.3774, 600.3719) (148.2662, 600.3398) (148.0834, 600.3077) (147.9451, 600.3077) knots 0 0 0 1 2 2 2
  spline S460 degree 2 poles (148.3922, 601.7576) (148.3872, 601.9132) (148.323, 602.1404) (148.2613, 602.217) knots 0 0 0 1 2 2 2
  spline S461 degree 2 poles (148.2613, 602.217) (148.1946, 602.3035) (147.9846, 602.3949) (147.829, 602.3949) knots 0 0 0 1 2 2 2
  spline S462 degree 2 poles (147.829, 602.3949) (147.6759, 602.3949) (147.461, 602.3035) (147.3721, 602.2145) knots 0 0 0 1 2 2 2
  spline S463 degree 2 poles (147.3721, 602.2145) (147.2856, 602.1232) (147.1967, 601.9033) (147.1843, 601.7576) knots 0 0 0 1 2 2 2
  line L444 (147.1843, 601.7576) -> (148.3922, 601.7576)
  line L445 (150.3707, 602.2343) -> (150.3509, 602.2343)
  spline S464 degree 2 poles (150.3509, 602.2343) (150.3064, 602.2467) (150.2101, 602.2516) (150.1434, 602.2516) knots 0 0 0 1 2 2 2
  spline S465 degree 2 poles (150.1434, 602.2516) (149.9878, 602.2516) (149.6815, 602.1157) (149.5432, 601.9824) knots 0 0 0 1 2 2 2
  line L446 (149.5432, 601.9824) -> (149.5432, 600.3596)
  line L447 (149.5432, 600.3596) -> (149.1579, 600.3596)
  line L448 (149.1579, 600.3596) -> (149.1579, 602.6468)
  line L449 (149.1579, 602.6468) -> (149.5432, 602.6468)
  line L450 (149.5432, 602.6468) -> (149.5432, 602.3059)
  spline S466 degree 2 poles (149.5432, 602.3059) (149.7532, 602.4937) (150.0669, 602.6468) (150.2151, 602.6468) knots 0 0 0 1 2 2 2
  spline S467 degree 2 poles (150.2151, 602.6468) (150.2743, 602.6468) (150.3336, 602.6419) (150.3707, 602.6344) knots 0 0 0 1 2 2 2
  line L451 (150.3707, 602.6344) -> (150.3707, 602.2343)
  line L452 (151.8798, 603.5434) -> (150.6868, 599.6976)
  line L453 (150.6868, 599.6976) -> (150.341, 599.6976)
  line L454 (150.341, 599.6976) -> (151.5291, 603.5434)
  line L455 (151.5291, 603.5434) -> (151.8798, 603.5434)
  line L456 (154.0312, 600.3596) -> (153.6459, 600.3596)
  line L457 (153.6459, 600.3596) -> (153.6459, 600.5917)
  spline S468 degree 2 poles (153.6459, 600.5917) (153.557, 600.5176) (153.4261, 600.4188) (153.3372, 600.3769) knots 0 0 0 1 2 2 2
  spline S469 degree 2 poles (153.3372, 600.3769) (153.2556, 600.3373) (153.0803, 600.2953) (152.9642, 600.2953) knots 0 0 0 1 2 2 2
  spline S470 degree 2 poles (152.9642, 600.2953) (152.7765, 600.2953) (152.4603, 600.451) (152.3491, 600.6016) knots 0 0 0 1 2 2 2
  spline S471 degree 2 poles (152.3491, 600.6016) (152.238, 600.7523) (152.1145, 601.1969) (152.1145, 601.4859) knots 0 0 0 1 2 2 2
  spline S472 degree 2 poles (152.1145, 601.4859) (152.1145, 601.7872) (152.2701, 602.2269) (152.406, 602.3924) knots 0 0 0 1 2 2 2
  spline S473 degree 2 poles (152.406, 602.3924) (152.5319, 602.5406) (152.8851, 602.711) (153.0803, 602.711) knots 0 0 0 1 2 2 2
  spline S474 degree 2 poles (153.0803, 602.711) (153.2507, 602.711) (153.5051, 602.6344) (153.6459, 602.5554) knots 0 0 0 1 2 2 2
  line L458 (153.6459, 602.5554) -> (153.6459, 603.5434)
  line L459 (153.6459, 603.5434) -> (154.0312, 603.5434)
  line L460 (154.0312, 603.5434) -> (154.0312, 600.3596)
  line L461 (153.6459, 600.9153) -> (153.6459, 602.2368)
  spline S475 degree 2 poles (153.6459, 602.2368) (153.5026, 602.3059) (153.2754, 602.3578) (153.1445, 602.3578) knots 0 0 0 1 2 2 2
  spline S476 degree 2 poles (153.1445, 602.3578) (152.8481, 602.3578) (152.5122, 601.9132) (152.5122, 601.4933) knots 0 0 0 1 2 2 2
  spline S477 degree 2 poles (152.5122, 601.4933) (152.5122, 601.0882) (152.7691, 600.6609) (153.0531, 600.6609) knots 0 0 0 1 2 2 2
  spline S478 degree 2 poles (153.0531, 600.6609) (153.2038, 600.6609) (153.5101, 600.7992) (153.6459, 600.9153) knots 0 0 0 1 2 2 2
  spline S479 degree 2 poles (156.5062, 601.5649) (156.5062, 600.9919) (155.9603, 600.3151) (155.5429, 600.3151) knots 0 0 0 1 2 2 2
  spline S480 degree 2 poles (155.5429, 600.3151) (155.3724, 600.3151) (155.1106, 600.3941) (154.9748, 600.4757) knots 0 0 0 1 2 2 2
  line L462 (154.9748, 600.4757) -> (154.9748, 599.5173)
  line L463 (154.9748, 599.5173) -> (154.5895, 599.5173)
  line L464 (154.5895, 599.5173) -> (154.5895, 602.6468)
  line L465 (154.5895, 602.6468) -> (154.9748, 602.6468)
  line L466 (154.9748, 602.6468) -> (154.9748, 602.4072)
  spline S481 degree 2 poles (154.9748, 602.4072) (155.118, 602.5381) (155.4688, 602.711) (155.6738, 602.711) knots 0 0 0 1 2 2 2
  spline S482 degree 2 poles (155.6738, 602.711) (156.0665, 602.711) (156.5062, 602.0886) (156.5062, 601.5649) knots 0 0 0 1 2 2 2
  spline S483 degree 2 poles (156.1085, 601.5205) (156.1085, 601.9132) (155.859, 602.3455) (155.5799, 602.3455) knots 0 0 0 1 2 2 2
  spline S484 degree 2 poles (155.5799, 602.3455) (155.4169, 602.3455) (155.1106, 602.1997) (154.9748, 602.0861) knots 0 0 0 1 2 2 2
  line L467 (154.9748, 602.0861) -> (154.9748, 600.7869)
  spline S485 degree 2 poles (154.9748, 600.7869) (155.1254, 600.7152) (155.3403, 600.6609) (155.4787, 600.6609) knots 0 0 0 1 2 2 2
  spline S486 degree 2 poles (155.4787, 600.6609) (155.7775, 600.6609) (156.1085, 601.1006) (156.1085, 601.5205) knots 0 0 0 1 2 2 2
  line L468 (158.1166, 603.5434) -> (156.9236, 599.6976)
  line L469 (156.9236, 599.6976) -> (156.5778, 599.6976)
  line L470 (156.5778, 599.6976) -> (157.7659, 603.5434)
  line L471 (157.7659, 603.5434) -> (158.1166, 603.5434)
  spline S487 degree 2 poles (160.6064, 601.2957) (160.6064, 601.0685) (160.4335, 600.7202) (160.2903, 600.6066) knots 0 0 0 1 2 2 2
  spline S488 degree 2 poles (160.2903, 600.6066) (160.1173, 600.4732) (159.7246, 600.3596) (159.4134, 600.3596) knots 0 0 0 1 2 2 2
  line L472 (159.4134, 600.3596) -> (158.539, 600.3596)
  line L473 (158.539, 600.3596) -> (158.539, 603.4076)
  line L474 (158.539, 603.4076) -> (159.3467, 603.4076)
  spline S489 degree 2 poles (159.3467, 603.4076) (159.6727, 603.4076) (159.9988, 603.3656) (160.147, 603.2841) knots 0 0 0 1 2 2 2
  spline S490 degree 2 poles (160.147, 603.2841) (160.3125, 603.1976) (160.4632, 602.9136) (160.4632, 602.7209) knots 0 0 0 1 2 2 2
  spline S491 degree 2 poles (160.4632, 602.7209) (160.4632, 602.506) (160.2359, 602.1651) (160.0358, 602.0688) knots 0 0 0 1 2 2 2
  line L475 (160.0358, 602.0688) -> (160.0358, 602.054)
  spline S492 degree 2 poles (160.0358, 602.054) (160.3075, 601.9799) (160.6064, 601.5872) (160.6064, 601.2957) knots 0 0 0 1 2 2 2
  spline S493 degree 2 poles (160.184, 601.2784) (160.184, 601.4513) (160.0852, 601.6736) (159.937, 601.7527) knots 0 0 0 1 2 2 2
  spline S494 degree 2 poles (159.937, 601.7527) (159.8407, 601.8021) (159.6135, 601.8317) (159.4035, 601.8317) knots 0 0 0 1 2 2 2
  line L476 (159.4035, 601.8317) -> (158.9441, 601.8317)
  line L477 (158.9441, 601.8317) -> (158.9441, 600.7054)
  line L478 (158.9441, 600.7054) -> (159.2726, 600.7054)
  spline S495 degree 2 poles (159.2726, 600.7054) (159.5394, 600.7054) (159.8456, 600.7548) (159.9642, 600.8338) knots 0 0 0 1 2 2 2
  spline S496 degree 2 poles (159.9642, 600.8338) (160.0778, 600.9153) (160.184, 601.1179) (160.184, 601.2784) knots 0 0 0 1 2 2 2
  spline S497 degree 2 poles (160.0408, 602.6641) (160.0408, 602.7728) (159.9667, 602.9358) (159.8852, 602.9827) knots 0 0 0 1 2 2 2
  spline S498 degree 2 poles (159.8852, 602.9827) (159.7864, 603.0371) (159.5468, 603.0618) (159.3319, 603.0618) knots 0 0 0 1 2 2 2
  line L479 (159.3319, 603.0618) -> (158.9441, 603.0618)
  line L480 (158.9441, 603.0618) -> (158.9441, 602.1701)
  line L481 (158.9441, 602.1701) -> (159.4035, 602.1701)
  spline S499 degree 2 poles (159.4035, 602.1701) (159.5937, 602.1701) (159.774, 602.2096) (159.8703, 602.2714) knots 0 0 0 1 2 2 2
  spline S500 degree 2 poles (159.8703, 602.2714) (159.9642, 602.3306) (160.0408, 602.5208) (160.0408, 602.6641) knots 0 0 0 1 2 2 2
  spline S501 degree 2 poles (162.8195, 601.8836) (162.8195, 601.0635) (162.3428, 600.2953) (161.8464, 600.2953) knots 0 0 0 1 2 2 2
  spline S502 degree 2 poles (161.8464, 600.2953) (161.3425, 600.2953) (160.8707, 601.0783) (160.8707, 601.8811) knots 0 0 0 1 2 2 2
  spline S503 degree 2 poles (160.8707, 601.8811) (160.8707, 602.7061) (161.3474, 603.4693) (161.8464, 603.4693) knots 0 0 0 1 2 2 2
  spline S504 degree 2 poles (161.8464, 603.4693) (162.3478, 603.4693) (162.8195, 602.6789) (162.8195, 601.8836) knots 0 0 0 1 2 2 2
  spline S505 degree 2 poles (162.2959, 600.9548) (162.3552, 601.1055) (162.4046, 601.5699) (162.4046, 601.8836) knots 0 0 0 1 2 2 2
  spline S506 degree 2 poles (162.4046, 601.8836) (162.4046, 602.1973) (162.3552, 602.6591) (162.2934, 602.8148) knots 0 0 0 1 2 2 2
  spline S507 degree 2 poles (162.2934, 602.8148) (162.2317, 602.9704) (162.0168, 603.1309) (161.8464, 603.1309) knots 0 0 0 1 2 2 2
  spline S508 degree 2 poles (161.8464, 603.1309) (161.6759, 603.1309) (161.4561, 602.9704) (161.3919, 602.8098) knots 0 0 0 1 2 2 2
  spline S509 degree 2 poles (161.3919, 602.8098) (161.3301, 602.6542) (161.2857, 602.18) (161.2857, 601.8811) knots 0 0 0 1 2 2 2
  spline S510 degree 2 poles (161.2857, 601.8811) (161.2857, 601.56) (161.3252, 601.1302) (161.3894, 600.9622) knots 0 0 0 1 2 2 2
  spline S511 degree 2 poles (161.3894, 600.9622) (161.4487, 600.8042) (161.6685, 600.6337) (161.8464, 600.6337) knots 0 0 0 1 2 2 2
  spline S512 degree 2 poles (161.8464, 600.6337) (162.0143, 600.6337) (162.2342, 600.7943) (162.2959, 600.9548) knots 0 0 0 1 2 2 2
  line L482 (165.1241, 602.9506) -> (163.8051, 600.3596)
  line L483 (163.8051, 600.3596) -> (163.3704, 600.3596)
  line L484 (163.3704, 600.3596) -> (164.7634, 603.0494)
  line L485 (164.7634, 603.0494) -> (163.19, 603.0494)
  line L486 (163.19, 603.0494) -> (163.19, 603.4076)
  line L487 (163.19, 603.4076) -> (165.1241, 603.4076)
  line L488 (165.1241, 603.4076) -> (165.1241, 602.9506)
  line L489 (167.4064, 603.0469) -> (165.9886, 603.0469)
  line L490 (165.9886, 603.0469) -> (165.9886, 602.1874)
  line L491 (165.9886, 602.1874) -> (167.3471, 602.1874)
  line L492 (167.3471, 602.1874) -> (167.3471, 601.8268)
  line L493 (167.3471, 601.8268) -> (165.9886, 601.8268)
  line L494 (165.9886, 601.8268) -> (165.9886, 600.3596)
  line L495 (165.9886, 600.3596) -> (165.5835, 600.3596)
  line L496 (165.5835, 600.3596) -> (165.5835, 603.4076)
  line L497 (165.5835, 603.4076) -> (167.4064, 603.4076)
  line L498 (167.4064, 603.4076) -> (167.4064, 603.0469)
  line L499 (169.4096, 600.3596) -> (167.9226, 600.3596)
  line L500 (167.9226, 600.3596) -> (167.9226, 600.6708)
  line L501 (167.9226, 600.6708) -> (168.4759, 600.6708)
  line L502 (168.4759, 600.6708) -> (168.4759, 602.7135)
  line L503 (168.4759, 602.7135) -> (167.9226, 602.7135)
  line L504 (167.9226, 602.7135) -> (167.9226, 602.9926)
  spline S513 degree 2 poles (167.9226, 602.9926) (168.2363, 602.9926) (168.5327, 603.1704) (168.5525, 603.4174) knots 0 0 0 1 2 2 2
  line L505 (168.5525, 603.4174) -> (168.8686, 603.4174)
  line L506 (168.8686, 603.4174) -> (168.8686, 600.6708)
  line L507 (168.8686, 600.6708) -> (169.4096, 600.6708)
  line L508 (169.4096, 600.6708) -> (169.4096, 600.3596)
  line L509 (172.2698, 600.3596) -> (171.8647, 600.3596)
  line L510 (171.8647, 600.3596) -> (171.8647, 601.8515)
  line L511 (171.8647, 601.8515) -> (170.4618, 601.8515)
  line L512 (170.4618, 601.8515) -> (170.4618, 600.3596)